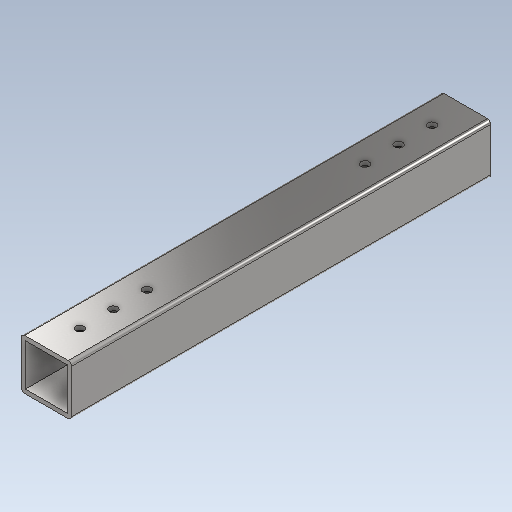
# Autodesk Inventor part: member_vertical
Saved by Autodesk Inventor 2021 (Build 250183000, 183)
## iProperties
Created: 2021-06-01
Part Number: member_vertical
Material: Steel, Galvanized
Document SubType Name: Modeling
Designer: Watchdog
Density: 7.85 g/cm^3
Appearance: Galvanized
Author: Watchdog
Autodesk Inventor part; units mm, degrees
ref_plane "YZ Plane" through (0, 0, 0) normal (1, 0, 0) x (0, 1, 0)
ref_plane "XZ Plane" through (0, 0, 0) normal (0, 1, 0) x (-1, 0, 0)
ref_plane "XY Plane" through (0, 0, 0) normal (0, 0, 1) x (1, 0, 0)
sketch "Sketch1" plane through (0, 0, 0) normal (0, 0, 1) x (1, 0, 0)
  line L0 (-15, 15) -> (15, 15)
  line L1 (15, 15) -> (15, -15)
  line L2 (15, -15) -> (-15, -15)
  line L3 (-15, -15) -> (-15, 15)
  line L4 (12.5, 12.5) -> (-12.5, 12.5)
  line L5 (-12.5, 12.5) -> (-12.5, -12.5)
  line L6 (-12.5, -12.5) -> (12.5, -12.5)
  line L7 (12.5, -12.5) -> (12.5, 12.5)
  point P0 (0, 0)
  dimension "d0" = 30
  dimension "d1" = 30
  dimension "d2" = 15
  dimension "d3" = 15
  dimension "d4" = 2.5
  constraints: 16 end point, 4 parallel, 2 perpendicular, 1 horizontal, 3 other
  measures "d0" distance of L0.start L0.end
  measures "d1" distance of L2.end L0.start
  measures "d2" distance from line of point (0, 0) L0
  measures "d3" distance from line of point (0, 0) L3
  measures "d4" distance between parallel lines of L0 L4
extrude "Extrusion1" add sketch "Sketch1" along normal blind 1000
fillet "Fillet1" radius 2 4 edges at (15, 15, 500) (-15, 15, 500) (-15, -15, 500) (15, -15, 500)
ref_plane "Work Plane1" through (0, 0, 250) normal (0, 0, -1) x (-1, 0, 0)
split "Split1" plane through (0, 0, 250) removes the side toward (0, 0, 1)
ref_plane "midPlane" through (-13, -15, 125) normal (0, 0, 1) x (1, 0, 0)
sketch "Sketch2" plane through (-13, 15, 0) normal (0, 1, 0) x (1, 0, 0)
  line L0 (0, -250) -> (26, -250) projected
  point P0 (13, 0)
  point P1 (13, -20)
  point P2 (13, -40)
  point P3 (13, -60)
  point P4 (13, -190)
  point P5 (13, -210)
  point P6 (13, -230)
  dimension "d9" = 0
  dimension "d10" = 0
  dimension "d11" = 0
  dimension "d12" = 0
  dimension "d13" = 0
  dimension "d14" = 0
  dimension "d15" = 20
  dimension "d16" = 20
  dimension "d17" = 20
  dimension "d18" = 20
  dimension "d19" = 20
  dimension "d20" = 20
  measures "d9" horizontal distance of point (13, 0) point (13, -20)
  measures "d10" horizontal distance of point (13, 0) point (13, -40)
  measures "d11" horizontal distance of point (13, 0) point (13, -60)
  measures "d12" horizontal distance of point (13, 0) point (13, -190)
  measures "d13" horizontal distance of point (13, 0) point (13, -210)
  measures "d14" horizontal distance of point (13, 0) point (13, -230)
  measures "d15" distance of point (13, 0) point (13, -20)
  measures "d16" distance of point (13, -20) point (13, -40)
  measures "d17" distance of point (13, -40) point (13, -60)
  measures "d18" distance from line of L0 point (13, -230)
  measures "d19" distance of point (13, -230) point (13, -210)
  measures "d20" distance of point (13, -210) point (13, -190)
hole "Hole1" at (0, 15, 20) at (0, 15, 40) at (0, 15, 60) at (0, 15, 190) at (0, 15, 210) at (0, 15, 230) direction (0, -1, 0) diameter 5 end through all
equation "\"d0\" = sm_varx_squareBarDimension"
equation "\"d1\" = d0"
equation "\"d2\" = 0.5 * d1"
equation "\"d3\" = 0.5 * d0"
equation "\"d4\" = sm_varx_squareBarThickness"
equation "\"d15\" = holeSpacing"
equation "\"d16\" = holeSpacing"
equation "\"d17\" = holeSpacing"
equation "\"d18\" = holeSpacing"
equation "\"d19\" = holeSpacing"
equation "\"d20\" = holeSpacing"
equation "\"d21\" = sm_varx_pinPlate_holeDiameter"
equation "\"hoop_angle_z\" = 45deg"
equation "\"hoop_bearing_length\" = 5deg"
equation "\"hoop_cable_diam\" = 5"
equation "\"hoop_cable_pulley_diam\" = 22"
equation "\"rack_tooth_addendum\" = 5"
equation "\"rack_tooth_dedendum\" = 5"
equation "\"rack_tooth_thickness\" = 5"
equation "\"secure_arm_angle\" = 35deg"
equation "\"secure_arm_radii\" = 9"
equation "\"support_baseClamp_platformLengthBuffer\" = 35"
equation "\"support_baseClamp_platformThickness\" = 15"
equation "\"support_baseClamp_platformWidthBuffer\" = 0"
equation "\"support_baseClamp_sleeveHoleDiameter\" = 12"
equation "\"support_baseClamp_sleeveSweepTerminationAngle\" = 55deg"
equation "\"support_baseClamp_thickness\" = 8"
equation "\"support_frame_endHoleBuffer\" = 25"
equation "\"support_frame_squareBarFillet\" = 2"
equation "\"support_frame_squareBarThickness\" = 5"
equation "\"hoop_tabs_thickness\" = 6"
equation "\"hoop_tabs_hole\" = 12"
equation "\"wheelchair_deployed_width\" = 635"
equation "\"wheelchair_deployed_length\" = 1067"
equation "\"wheelchair_deployed_height\" = 914"
equation "\"sm_varx_squareBarDimension\" = 30"
equation "\"sm_varx_squareBarThickness\" = 2.5"
equation "\"sm_varx_member_tolerance\" = 0.5"
equation "\"sm_varx_pinPlate_thickness\" = 5"
equation "\"sm_varx_pinPlate_holeDiameter\" = 5"
equation "\"holeSpacing\" = 20"
body "Solid1"
